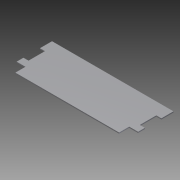
# Autodesk Inventor part: ElectronicsBoardVerticalBottomDropped
Saved by Autodesk Inventor 2012 (Build 160160000, 160)
## iProperties
Created: 2012-01-10
Part Number: ElectronicsBoardVerticalBottomDropped
Material: Default
Document SubType Name: Modeling
Designer: William
Density: 1 g/cm^3
Author: William
Autodesk Inventor part; units mm, degrees
ref_plane "YZ Plane" through (0, 0, 0) normal (1, 0, 0) x (0, 1, 0)
ref_plane "XZ Plane" through (0, 0, 0) normal (0, 1, 0) x (-1, 0, 0)
ref_plane "XY Plane" through (0, 0, 0) normal (0, 0, 1) x (1, 0, 0)
sketch "Sketch1" plane through (0, 0, 0) normal (0, 0, 1) x (1, 0, 0)
  line L0 (185.4498, -59.7201) -> (-424.1502, -59.7201)
  line L1 (-424.1502, -59.7201) -> (-424.1502, -54.6401)
  line L2 (-424.1502, -54.6401) -> (185.4498, -54.6401)
  line L3 (185.4498, -54.6401) -> (185.4498, -59.7201)
  point P0 (0, 0)
  dimension "d0" = 609.6
  dimension "d1" = 5.08
  constraints: 8 end point, 2 parallel, 1 horizontal, 1 perpendicular
  measures "d0" distance of L1.end L2.end
  measures "d1" distance of L0.end L1.end
extrude "Extrusion1" add sketch "Sketch1" along normal blind 228.6
sketch "Sketch2" plane through (-424.1502, -59.7201, 0) normal (0, -1, 0) x (1, 0, 0)
  line L0 (0, 0) -> (0, 228.6) projected
  line L1 (609.6, 0) -> (0, 0) projected
  line L2 (609.6, 0) -> (609.6, 228.6) projected
  line L3 (0, 228.6) -> (44.45, 228.6)
  line L4 (44.45, 228.6) -> (44.45, 177.8)
  line L5 (44.45, 177.8) -> (0, 177.8)
  line L6 (0, 177.8) -> (0, 228.6)
  line L7 (609.6, 228.6) -> (565.15, 228.6)
  line L8 (565.15, 228.6) -> (565.15, 177.8)
  line L9 (565.15, 177.8) -> (609.6, 177.8)
  line L10 (609.6, 177.8) -> (609.6, 228.6)
  line L11 (609.6, 60.96) -> (584.2, 60.96)
  line L12 (584.2, 60.96) -> (584.2, 143.51)
  line L13 (584.2, 143.51) -> (609.6, 143.51)
  line L14 (609.6, 143.51) -> (609.6, 60.96)
  line L15 (0, 60.96) -> (25.4, 60.96)
  line L16 (25.4, 60.96) -> (25.4, 143.51)
  line L17 (25.4, 143.51) -> (0, 143.51)
  line L18 (0, 143.51) -> (0, 60.96)
  point P0 (424.1502, 0)
  dimension "d4" = 44.45
  dimension "d5" = 50.8
  dimension "d6" = 44.45
  dimension "d7" = 50.8
  dimension "d8" = 60.96
  dimension "d9" = 60.96
  dimension "d10" = 25.4
  dimension "d11" = 25.4
  dimension "d12" = 82.55
  dimension "d13" = 82.55
  constraints: 32 end point, 8 parallel, 4 horizontal, 4 perpendicular, 2 point on line
  measures "d4" distance of L4.end L5.end
  measures "d5" distance of L3.end L4.end
  measures "d6" distance of L9.end L8.end
  measures "d7" distance of L8.end L7.end
  measures "d8" distance between parallel lines of L1 L15
  measures "d9" distance between parallel lines of L1 L11
  measures "d10" distance between parallel lines of L14 L12
  measures "d11" distance between parallel lines of L18 L16
  measures "d12" distance between parallel lines of L15 L17
  measures "d13" distance of L11.end L12.end
extrude "Extrusion2" cut sketch "Sketch2" against normal blind 25.4
equation "\"d6\" = d4"
equation "\"d7\" = d5"
equation "\"d9\" = d8"
equation "\"d10\" = d11"
equation "\"d13\" = d12"
body "Solid1"
